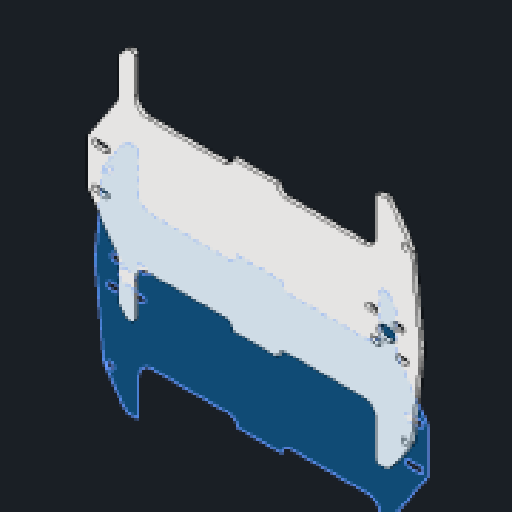
# Autodesk Inventor part: Aluminium Plate
Saved by Autodesk Inventor 2023.2 (Build 272271030, 271C)
## iProperties
Created: 2024-02-26
Part Number: Aluminium Plate
Material: Aluminum 6061
Document SubType Name: Modeling
Designer: robpl
Mass: 7.61954 g
Surface Area: 47.9052 cm^2
Volume: 2.82205 cm^3
Density: 2.7 g/cm^3
Appearance: Aluminum - Flat
Author: robpl
Autodesk Inventor part; units mm, degrees
ref_plane "YZ Plane" through (0, 0, 0) normal (1, 0, 0) x (0, 1, 0)
ref_plane "XZ Plane" through (0, 0, 0) normal (0, 1, 0) x (-1, 0, 0)
ref_plane "XY Plane" through (0, 0, 0) normal (0, 0, 1) x (1, 0, 0)
sketch "Sketch1" plane through (0, 0, 0) normal (0, 0, 1) x (1, 0, 0)
  arc A0 (49.1621, -12) -> (49.9853, -11.6297) centre (49.1621, -10.9) ccw projected
  arc A1 (49.9853, -11.6297) -> (61.3442, 6.3785) centre (0.77, 32) ccw projected
  arc A2 (61.3442, 6.3785) -> (60.2122, 9.0273) centre (59.5022, 7.1576) ccw projected
  arc A3 (61.2196, 14.348) -> (60.2122, 9.0273) centre (61.1884, 11.5982) ccw projected
  arc A4 (61.2196, 14.348) -> (63.2363, 16.5025) centre (61.2423, 16.3479) ccw projected
  line L0 (63.2363, 16.5025) -> (62.0377, 31.9587) projected
  line L1 (62.0377, 31.9587) -> (63.3538, 47.486) projected
  arc A5 (63.3538, 47.486) -> (61.2883, 49.6536) centre (61.3609, 47.6549) ccw projected
  arc A6 (60.2122, 54.9727) -> (61.2883, 49.6536) centre (61.1884, 52.4018) ccw projected
  arc A7 (60.2122, 54.9727) -> (61.3442, 57.6215) centre (59.5022, 56.8424) ccw projected
  arc A8 (61.3442, 57.6215) -> (49.9853, 75.6297) centre (0.77, 32) ccw projected
  arc A9 (49.9853, 75.6297) -> (49.1621, 76) centre (49.1621, 74.9) ccw projected
  line L2 (46.6, 76) -> (49.1621, 76) projected
  arc A10 (46.6, 76) -> (45.5, 74.9) centre (46.6, 74.9) ccw projected
  line L3 (45.5, 62) -> (45.5, 74.9) projected
  arc A11 (40.5, 57) -> (45.5, 62) centre (40.5, 62) ccw projected
  line L4 (11.3595, 57) -> (40.5, 57) projected
  arc A12 (8.3595, 60) -> (11.3595, 57) centre (11.3595, 60) ccw projected
  line L5 (-8.3595, 60) -> (8.3595, 60) projected
  arc A13 (-11.3595, 57) -> (-8.3595, 60) centre (-11.3595, 60) ccw projected
  line L6 (-40.5, 57) -> (-11.3595, 57) projected
  arc A14 (-45.5, 62) -> (-40.5, 57) centre (-40.5, 62) ccw projected
  line L7 (-45.5, 74.9) -> (-45.5, 62) projected
  arc A15 (-45.5, 74.9) -> (-46.6, 76) centre (-46.6, 74.9) ccw projected
  line L8 (-47.6221, 76) -> (-46.6, 76) projected
  arc A16 (-47.6221, 76) -> (-48.4453, 75.6297) centre (-47.6221, 74.9) ccw projected
  arc A17 (-48.4453, 75.6297) -> (-50.9534, 72.6248) centre (0.77, 32) ccw projected
  arc A18 (-50.9534, 72.6248) -> (-51.1884, 71.9454) centre (-50.0884, 71.9454) ccw projected
  line L9 (-51.1884, 71.9454) -> (-51.1884, 59.7084) projected
  arc A19 (-52.0225, 56.9433) -> (-51.1884, 59.7084) centre (-56.1884, 59.7084) ccw projected
  line L10 (-52.0225, 56.9433) -> (-62.4995, 41.1591) projected
  arc A20 (-62.4995, 41.1591) -> (-63, 39.5) centre (-60, 39.5) ccw projected
  line L11 (-63, 39.5) -> (-63, 24.5) projected
  arc A21 (-63, 24.5) -> (-62.4995, 22.8409) centre (-60, 24.5) ccw projected
  line L12 (-62.4995, 22.8409) -> (-52.0225, 7.0567) projected
  arc A22 (-51.1884, 4.2916) -> (-52.0225, 7.0567) centre (-56.1884, 4.2916) ccw projected
  line L13 (-51.1884, 4.2916) -> (-51.1884, -7.9454) projected
  arc A23 (-51.1884, -7.9454) -> (-50.9534, -8.6248) centre (-50.0884, -7.9454) ccw projected
  arc A24 (-50.9534, -8.6248) -> (-48.4453, -11.6297) centre (0.77, 32) ccw projected
  arc A25 (-48.4453, -11.6297) -> (-47.6221, -12) centre (-47.6221, -10.9) ccw projected
  line L14 (-46.6, -12) -> (-47.6221, -12) projected
  arc A26 (-46.6, -12) -> (-45.5, -10.9) centre (-46.6, -10.9) ccw projected
  line L15 (-45.5, 2) -> (-45.5, -10.9) projected
  arc A27 (-40.5, 7) -> (-45.5, 2) centre (-40.5, 2) ccw projected
  line L16 (-11.3595, 7) -> (-40.5, 7) projected
  arc A28 (-8.3595, 4) -> (-11.3595, 7) centre (-11.3595, 4) ccw projected
  line L17 (-8.3595, 4) -> (8.3595, 4) projected
  arc A29 (11.3595, 7) -> (8.3595, 4) centre (11.3595, 4) ccw projected
  line L18 (40.5, 7) -> (11.3595, 7) projected
  arc A30 (45.5, 2) -> (40.5, 7) centre (40.5, 2) ccw projected
  line L19 (45.5, -10.9) -> (45.5, 2) projected
  arc A31 (45.5, -10.9) -> (46.6, -12) centre (46.6, -10.9) ccw projected
  line L20 (49.1621, -12) -> (46.6, -12) projected
  line L21 (56.1569, 23.8431) -> (54.1569, 23.8431) projected
  arc A32 (54.1569, 28.8431) -> (54.1569, 23.8431) centre (54.1569, 26.3431) ccw projected
  line L22 (54.1569, 28.8431) -> (56.1569, 28.8431) projected
  arc A33 (56.1569, 23.8431) -> (56.1569, 28.8431) centre (56.1569, 26.3431) ccw projected
  line L23 (42.8431, 40.1569) -> (44.8431, 40.1569) projected
  arc A34 (44.8431, 35.1569) -> (44.8431, 40.1569) centre (44.8431, 37.6569) ccw projected
  line L24 (44.8431, 35.1569) -> (42.8431, 35.1569) projected
  arc A35 (42.8431, 40.1569) -> (42.8431, 35.1569) centre (42.8431, 37.6569) ccw projected
  arc A36 (45.0797, 30.2574) -> (46.0569, 31.4695) centre (45.0797, 31.2574) ccw projected
  arc A37 (48.5, 34.5) -> (46.0569, 31.4695) centre (48.5, 32) ccw projected
  line L25 (48.5, 34.5) -> (49.3223, 34.5) projected
  arc A38 (49.3223, 34.5) -> (50.2996, 35.7122) centre (49.3223, 35.5) ccw projected
  arc A39 (52.7426, 38.7426) -> (50.2996, 35.7122) centre (52.7426, 36.2426) ccw projected
  line L26 (52.7426, 38.7426) -> (54.7426, 38.7426) projected
  arc A40 (54.7426, 33.7426) -> (54.7426, 38.7426) centre (54.7426, 36.2426) ccw projected
  line L27 (54.7426, 33.7426) -> (53.9203, 33.7426) projected
  arc A41 (53.9203, 33.7426) -> (52.9431, 32.5305) centre (53.9203, 32.7426) ccw projected
  arc A42 (50.5, 29.5) -> (52.9431, 32.5305) centre (50.5, 32) ccw projected
  line L28 (50.5, 29.5) -> (49.6777, 29.5) projected
  arc A43 (49.6777, 29.5) -> (48.7004, 28.2878) centre (49.6777, 28.5) ccw projected
  arc A44 (46.2574, 25.2574) -> (48.7004, 28.2878) centre (46.2574, 27.7574) ccw projected
  line L29 (46.2574, 25.2574) -> (44.2574, 25.2574) projected
  arc A45 (44.2574, 30.2574) -> (44.2574, 25.2574) centre (44.2574, 27.7574) ccw projected
  line L30 (44.2574, 30.2574) -> (45.0797, 30.2574) projected
  arc A46 (-56, 22) -> (-56, 27) centre (-56, 24.5) ccw projected
  line L31 (-56, 22) -> (-60, 22) projected
  arc A47 (-60, 27) -> (-60, 22) centre (-60, 24.5) ccw projected
  line L32 (-60, 27) -> (-56, 27) projected
  line L33 (-56, 37) -> (-60, 37) projected
  arc A48 (-60, 42) -> (-60, 37) centre (-60, 39.5) ccw projected
  line L34 (-60, 42) -> (-56, 42) projected
  arc A49 (-56, 37) -> (-56, 42) centre (-56, 39.5) ccw projected
  arc A50 (63.4897, 12.2028) -> (63.5375, 12.619) centre (62.4407, 12.5339) ccw projected
  line L35 (63.5375, 12.619) -> (63.2363, 16.5025) projected
  arc A51 (61.2196, 14.348) -> (63.2363, 16.5025) centre (61.2423, 16.3479) ccw projected
  arc A52 (61.2196, 14.348) -> (60.2122, 9.0273) centre (61.1884, 11.5982) ccw projected
  arc A53 (61.3442, 6.3785) -> (60.2122, 9.0273) centre (59.5022, 7.1576) ccw projected
  arc A54 (61.3442, 6.3785) -> (63.4897, 12.2028) centre (0.77, 32) ccw projected
  circle A55 centre (61.1884, 11.5982) radius 1.25 projected
  circle A56 centre (61.1884, 52.4018) radius 1.25 projected
  arc A57 (63.652, 51.0045) -> (63.6069, 51.4222) centre (62.5559, 51.0974) ccw projected
  arc A58 (63.6069, 51.4222) -> (61.3442, 57.6215) centre (0.77, 32) ccw projected
  arc A59 (60.2122, 54.9727) -> (61.3442, 57.6215) centre (59.5022, 56.8424) ccw projected
  arc A60 (60.2122, 54.9727) -> (61.2883, 49.6536) centre (61.1884, 52.4018) ccw projected
  arc A61 (63.3538, 47.486) -> (61.2883, 49.6536) centre (61.3609, 47.6549) ccw projected
  line L36 (63.3538, 47.486) -> (63.652, 51.0045) projected
  line L37 (54.7426, 37.4926) -> (52.7426, 37.4926) projected
  arc A62 (54.7426, 34.9926) -> (54.7426, 37.4926) centre (54.7426, 36.2426) ccw projected
  line L38 (52.7426, 34.9926) -> (54.7426, 34.9926) projected
  arc A63 (52.7426, 37.4926) -> (52.7426, 34.9926) centre (52.7426, 36.2426) ccw projected
  arc A64 (52.9431, 32.5305) -> (50.5, 34.5) centre (50.5, 32) ccw projected
  arc A65 (53.9203, 33.7426) -> (52.9431, 32.5305) centre (53.9203, 32.7426) ccw projected
  line L39 (54.7426, 33.7426) -> (53.9203, 33.7426) projected
  arc A66 (54.7426, 33.7426) -> (54.7426, 38.7426) centre (54.7426, 36.2426) ccw projected
  line L40 (52.7426, 38.7426) -> (54.7426, 38.7426) projected
  arc A67 (52.7426, 38.7426) -> (50.2996, 35.7122) centre (52.7426, 36.2426) ccw projected
  arc A68 (49.3223, 34.5) -> (50.2996, 35.7122) centre (49.3223, 35.5) ccw projected
  line L41 (49.3223, 34.5) -> (50.5, 34.5) projected
  arc A69 (46.0569, 31.4695) -> (48.5, 29.5) centre (48.5, 32) ccw projected
  arc A70 (45.0797, 30.2574) -> (46.0569, 31.4695) centre (45.0797, 31.2574) ccw projected
  line L42 (44.2574, 30.2574) -> (45.0797, 30.2574) projected
  arc A71 (44.2574, 30.2574) -> (44.2574, 25.2574) centre (44.2574, 27.7574) ccw projected
  line L43 (46.2574, 25.2574) -> (44.2574, 25.2574) projected
  arc A72 (46.2574, 25.2574) -> (48.7004, 28.2878) centre (46.2574, 27.7574) ccw projected
  arc A73 (49.6777, 29.5) -> (48.7004, 28.2878) centre (49.6777, 28.5) ccw projected
  line L44 (49.6777, 29.5) -> (48.5, 29.5) projected
  line L45 (46.2574, 29.0074) -> (44.2574, 29.0074) projected
  arc A74 (46.2574, 26.5074) -> (46.2574, 29.0074) centre (46.2574, 27.7574) ccw projected
  line L46 (44.2574, 26.5074) -> (46.2574, 26.5074) projected
  arc A75 (44.2574, 29.0074) -> (44.2574, 26.5074) centre (44.2574, 27.7574) ccw projected
  arc A76 (54.1569, 28.8431) -> (54.1569, 23.8431) centre (54.1569, 26.3431) ccw projected
  line L47 (56.1569, 23.8431) -> (54.1569, 23.8431) projected
  arc A77 (56.1569, 23.8431) -> (56.1569, 28.8431) centre (56.1569, 26.3431) ccw projected
  line L48 (54.1569, 28.8431) -> (56.1569, 28.8431) projected
  line L49 (56.1569, 27.5931) -> (54.1569, 27.5931) projected
  arc A78 (56.1569, 25.0931) -> (56.1569, 27.5931) centre (56.1569, 26.3431) ccw projected
  line L50 (54.1569, 25.0931) -> (56.1569, 25.0931) projected
  arc A79 (54.1569, 27.5931) -> (54.1569, 25.0931) centre (54.1569, 26.3431) ccw projected
  arc A80 (44.8431, 35.1569) -> (44.8431, 40.1569) centre (44.8431, 37.6569) ccw projected
  line L51 (42.8431, 40.1569) -> (44.8431, 40.1569) projected
  arc A81 (42.8431, 40.1569) -> (42.8431, 35.1569) centre (42.8431, 37.6569) ccw projected
  line L52 (44.8431, 35.1569) -> (42.8431, 35.1569) projected
  line L53 (44.8431, 38.9069) -> (42.8431, 38.9069) projected
  arc A82 (44.8431, 36.4069) -> (44.8431, 38.9069) centre (44.8431, 37.6569) ccw projected
  line L54 (42.8431, 36.4069) -> (44.8431, 36.4069) projected
  arc A83 (42.8431, 38.9069) -> (42.8431, 36.4069) centre (42.8431, 37.6569) ccw projected
  line L55 (-56, 22) -> (-60, 22) projected
  arc A84 (-56, 22) -> (-56, 27) centre (-56, 24.5) ccw projected
  line L56 (-60, 27) -> (-56, 27) projected
  arc A85 (-60, 27) -> (-60, 22) centre (-60, 24.5) ccw projected
  line L57 (-60, 23.25) -> (-56, 23.25) projected
  arc A86 (-60, 25.75) -> (-60, 23.25) centre (-60, 24.5) ccw projected
  line L58 (-56, 25.75) -> (-60, 25.75) projected
  arc A87 (-56, 23.25) -> (-56, 25.75) centre (-56, 24.5) ccw projected
  arc A88 (-60, 42) -> (-60, 37) centre (-60, 39.5) ccw projected
  line L59 (-56, 37) -> (-60, 37) projected
  arc A89 (-56, 37) -> (-56, 42) centre (-56, 39.5) ccw projected
  line L60 (-60, 42) -> (-56, 42) projected
  line L61 (-60, 38.25) -> (-56, 38.25) projected
  arc A90 (-60, 40.75) -> (-60, 38.25) centre (-60, 39.5) ccw projected
  line L62 (-56, 40.75) -> (-60, 40.75) projected
  arc A91 (-56, 38.25) -> (-56, 40.75) centre (-56, 39.5) ccw projected
  point P0 (0, 0)
  point P1 (56.9489, 66.3148)
  point P2 (58.8517, 62.9872)
  point P3 (60.925, 8.5632)
  point P4 (62.8417, 15.1472)
  point P5 (56.9489, -2.3148)
  point P6 (58.8283, 1.0982)
  point P7 (58.6807, 0.8224)
  point P8 (58.7883, 1.2239)
  point P9 (56.8648, -2.3375)
extrude "Extrusion1" add sketch "Sketch1" along normal blind 1.6 contours L20 A31 L19 A30 L18 A29 L17 A28 L16 A27 L15 A26 L14 A25 A24 A23 L13 A22 L12 A21 L11 A20 L10 A19 L9 A18 A17 A16 L8 A15 L7 A14 L6 A13 L5 A12 L4 A11 L3 A10 L2 A9 A8 A7 A6 A5 L1 L0 A4 A3 A2 A1 A0 | A2 A3 A4 L35 A50 A54 | A5 A6 A7 A58 A57 L36 | L21 A32 L22 A33 | L23 A34 L24 A35 | A36 A69 L44 A43 A44 L29 A45 L30 | A38 A39 L26 A40 L27 A41 A64 L41 | L31 A47 L32 A46 | L33 A48 L34 A49
sketch "Sketch3" plane through (0, 0, 1.6) normal (0, 0, 1) x (1, 0, 0)
  arc A0 (49.9853, 75.6297) -> (49.1621, 76) centre (49.1621, 74.9) ccw projected
  line L0 (49.1621, 76) -> (46.6, 76) projected
  arc A1 (46.6, 76) -> (45.5, 74.9) centre (46.6, 74.9) ccw projected
  line L1 (45.5, 74.9) -> (45.5, 62) projected
  arc A2 (40.5, 57) -> (45.5, 62) centre (40.5, 62) ccw projected
  line L2 (40.5, 57) -> (11.3595, 57) projected
  arc A3 (8.3595, 60) -> (11.3595, 57) centre (11.3595, 60) ccw projected
  line L3 (8.3595, 60) -> (-8.3595, 60) projected
  arc A4 (-11.3595, 57) -> (-8.3595, 60) centre (-11.3595, 60) ccw projected
  line L4 (-11.3595, 57) -> (-40.5, 57) projected
  arc A5 (-45.5, 62) -> (-40.5, 57) centre (-40.5, 62) ccw projected
  line L5 (-45.5, 62) -> (-45.5, 74.9) projected
  arc A6 (-45.5, 74.9) -> (-46.6, 76) centre (-46.6, 74.9) ccw projected
  line L6 (-46.6, 76) -> (-47.6221, 76) projected
  arc A7 (-47.6221, 76) -> (-48.4453, 75.6297) centre (-47.6221, 74.9) ccw projected
  arc A8 (-48.4453, 75.6297) -> (-50.9534, 72.6248) centre (0.77, 32) ccw projected
  arc A9 (-50.9534, 72.6248) -> (-51.1884, 71.9454) centre (-50.0884, 71.9454) ccw projected
  line L7 (-51.1884, 71.9454) -> (-51.1884, 59.7084) projected
  arc A10 (-52.0225, 56.9433) -> (-51.1884, 59.7084) centre (-56.1884, 59.7084) ccw projected
  line L8 (-52.0225, 56.9433) -> (-62.4995, 41.1591) projected
  arc A11 (-62.4995, 41.1591) -> (-63, 39.5) centre (-60, 39.5) ccw projected
  line L9 (-63, 39.5) -> (-63, 24.5) projected
  arc A12 (-63, 24.5) -> (-62.4995, 22.8409) centre (-60, 24.5) ccw projected
  line L10 (-62.4995, 22.8409) -> (-52.0225, 7.0567) projected
  arc A13 (-51.1884, 4.2916) -> (-52.0225, 7.0567) centre (-56.1884, 4.2916) ccw projected
  line L11 (-51.1884, 4.2916) -> (-51.1884, -7.9454) projected
  arc A14 (-51.1884, -7.9454) -> (-50.9534, -8.6248) centre (-50.0884, -7.9454) ccw projected
  arc A15 (-50.9534, -8.6248) -> (-48.4453, -11.6297) centre (0.77, 32) ccw projected
  arc A16 (-48.4453, -11.6297) -> (-47.6221, -12) centre (-47.6221, -10.9) ccw projected
  line L12 (-47.6221, -12) -> (-46.6, -12) projected
  arc A17 (-46.6, -12) -> (-45.5, -10.9) centre (-46.6, -10.9) ccw projected
  line L13 (-45.5, -10.9) -> (-45.5, 2) projected
  arc A18 (-40.5, 7) -> (-45.5, 2) centre (-40.5, 2) ccw projected
  line L14 (-40.5, 7) -> (-11.3595, 7) projected
  arc A19 (-8.3595, 4) -> (-11.3595, 7) centre (-11.3595, 4) ccw projected
  line L15 (-8.3595, 4) -> (8.3595, 4) projected
  arc A20 (11.3595, 7) -> (8.3595, 4) centre (11.3595, 4) ccw projected
  line L16 (11.3595, 7) -> (40.5, 7) projected
  arc A21 (45.5, 2) -> (40.5, 7) centre (40.5, 2) ccw projected
  line L17 (45.5, 2) -> (45.5, -10.9) projected
  arc A22 (45.5, -10.9) -> (46.6, -12) centre (46.6, -10.9) ccw projected
  line L18 (46.6, -12) -> (49.1621, -12) projected
  arc A23 (49.1621, -12) -> (49.9853, -11.6297) centre (49.1621, -10.9) ccw projected
  arc A24 (49.9853, -11.6297) -> (63.4897, 12.2028) centre (0.77, 32) ccw projected
  arc A25 (63.4897, 12.2028) -> (63.5375, 12.619) centre (62.4407, 12.5339) ccw projected
  line L19 (63.5375, 12.619) -> (62.0377, 31.9587) projected
  line L20 (62.0377, 31.9587) -> (63.652, 51.0045) projected
  arc A26 (63.652, 51.0045) -> (63.6069, 51.4222) centre (62.5559, 51.0974) ccw projected
  arc A27 (63.6069, 51.4222) -> (49.9853, 75.6297) centre (0.77, 32) ccw projected
  arc A28 (44.8431, 36.4069) -> (44.8431, 38.9069) centre (44.8431, 37.6569) ccw projected
  line L21 (44.8431, 36.4069) -> (42.8431, 36.4069) projected
  arc A29 (42.8431, 38.9069) -> (42.8431, 36.4069) centre (42.8431, 37.6569) ccw projected
  line L22 (42.8431, 38.9069) -> (44.8431, 38.9069) projected
  arc A30 (56.1569, 25.0931) -> (56.1569, 27.5931) centre (56.1569, 26.3431) ccw projected
  line L23 (56.1569, 25.0931) -> (54.1569, 25.0931) projected
  arc A31 (54.1569, 27.5931) -> (54.1569, 25.0931) centre (54.1569, 26.3431) ccw projected
  line L24 (54.1569, 27.5931) -> (56.1569, 27.5931) projected
  arc A32 (-60, 25.75) -> (-60, 23.25) centre (-60, 24.5) ccw projected
  line L25 (-60, 25.75) -> (-56, 25.75) projected
  arc A33 (-56, 23.25) -> (-56, 25.75) centre (-56, 24.5) ccw projected
  line L26 (-56, 23.25) -> (-60, 23.25) projected
  arc A34 (-60, 40.75) -> (-60, 38.25) centre (-60, 39.5) ccw projected
  line L27 (-60, 40.75) -> (-56, 40.75) projected
  arc A35 (-56, 38.25) -> (-56, 40.75) centre (-56, 39.5) ccw projected
  line L28 (-56, 38.25) -> (-60, 38.25) projected
  circle A36 centre (61.1884, 52.4018) radius 1.25 projected
  circle A37 centre (61.1884, 11.5982) radius 1.25 projected
  arc A38 (46.2574, 26.5074) -> (46.2574, 29.0074) centre (46.2574, 27.7574) ccw projected
  line L29 (46.2574, 26.5074) -> (44.2574, 26.5074) projected
  arc A39 (44.2574, 29.0074) -> (44.2574, 26.5074) centre (44.2574, 27.7574) ccw projected
  line L30 (44.2574, 29.0074) -> (46.2574, 29.0074) projected
  arc A40 (50.5, 29.5) -> (50.5, 34.5) centre (50.5, 32) ccw projected
  line L31 (50.5, 29.5) -> (48.5, 29.5) projected
  arc A41 (48.5, 34.5) -> (48.5, 29.5) centre (48.5, 32) ccw projected
  line L32 (48.5, 34.5) -> (50.5, 34.5) projected
  arc A42 (54.7426, 34.9926) -> (54.7426, 37.4926) centre (54.7426, 36.2426) ccw projected
  line L33 (54.7426, 34.9926) -> (52.7426, 34.9926) projected
  arc A43 (52.7426, 37.4926) -> (52.7426, 34.9926) centre (52.7426, 36.2426) ccw projected
  line L34 (52.7426, 37.4926) -> (54.7426, 37.4926) projected
  line L35 (50.5, -2.9274) -> (50.5, 2)
  arc A44 (50.5, 2) -> (40.5, 12) centre (40.5, 2) ccw
  line L36 (40.5, 12) -> (11.3595, 12)
  arc A45 (11.3595, 12) -> (5.1145, 9) centre (11.3595, 4) ccw
  line L37 (5.1145, 9) -> (-5.1145, 9)
  arc A46 (-5.1145, 9) -> (-11.3595, 12) centre (-11.3595, 4) ccw
  line L38 (-11.3595, 12) -> (-40.5, 12)
  arc A47 (-40.5, 12) -> (-46.1884, 10.2245) centre (-40.5, 2) ccw
  line L39 (-46.1884, 10.2245) -> (-46.1884, 4.2916)
  arc A48 (-46.1884, 4.2916) -> (-47.8567, 9.8219) centre (-56.1884, 4.2916) ccw
  line L40 (-47.8567, 9.8219) -> (-58, 25.1034)
  line L41 (-58, 25.1034) -> (-58, 38.8966)
  line L42 (-58, 38.8966) -> (-47.8567, 54.1781)
  arc A49 (-47.8567, 54.1781) -> (-46.1884, 59.7084) centre (-56.1884, 59.7084) ccw
  line L43 (-46.1884, 59.7084) -> (-46.1884, 53.7755)
  arc A50 (-46.1884, 53.7755) -> (-40.5, 52) centre (-40.5, 62) ccw
  line L44 (-40.5, 52) -> (-11.3595, 52)
  arc A51 (-11.3595, 52) -> (-5.1145, 55) centre (-11.3595, 60) ccw
  line L45 (-5.1145, 55) -> (5.1145, 55)
  arc A52 (5.1145, 55) -> (11.3595, 52) centre (11.3595, 60) ccw
  line L46 (11.3595, 52) -> (40.5, 52)
  arc A53 (40.5, 52) -> (50.5, 62) centre (40.5, 62) ccw
  line L47 (50.5, 62) -> (50.5, 66.9274)
  arc A54 (58.6047, 50.6584) -> (50.5, 66.9274) centre (0.77, 32) ccw
  line L48 (58.6047, 50.6584) -> (57.0213, 31.9766)
  line L49 (57.0213, 31.9766) -> (58.493, 12.9987)
  arc A55 (50.5, -2.9274) -> (58.493, 12.9987) centre (0.77, 32) ccw
  line L50 (11.3595, 52) -> (8.3595, 52)
  line L51 (8.3595, 52) -> (-11.3595, 52)
  arc A56 (8.3595, 60) -> (11.3595, 57) centre (11.3595, 60) ccw projected
  line L52 (11.3595, 57) -> (-11.3595, 57)
  arc A57 (11.3595, 7) -> (8.3595, 4) centre (11.3595, 4) ccw projected
  line L53 (11.3595, 7) -> (-11.3595, 7)
  line L54 (11.3595, 12) -> (-11.3595, 12)
  circle A58 centre (61.1884, 11.5982) radius 3
  circle A59 centre (61.1884, 52.4018) radius 3
  line L55 (42.8431, 34.4069) -> (44.8431, 34.4069)
  arc A60 (44.8431, 34.4069) -> (44.8431, 40.9069) centre (44.8431, 37.6569) ccw
  line L56 (44.8431, 40.9069) -> (42.8431, 40.9069)
  arc A61 (42.8431, 40.9069) -> (42.8431, 34.4069) centre (42.8431, 37.6569) ccw
  arc A62 (46.2574, 24.5074) -> (46.2574, 31.0074) centre (46.2574, 27.7574) ccw
  line L57 (46.2574, 24.5074) -> (44.2574, 24.5074)
  arc A63 (44.2574, 31.0074) -> (44.2574, 24.5074) centre (44.2574, 27.7574) ccw
  line L58 (44.2574, 31.0074) -> (46.2574, 31.0074)
  line L59 (48.5, 27.5) -> (50.5, 27.5)
  arc A64 (50.5, 27.5) -> (50.5, 36.5) centre (50.5, 32) ccw
  line L60 (50.5, 36.5) -> (48.5, 36.5)
  arc A65 (48.5, 36.5) -> (48.5, 27.5) centre (48.5, 32) ccw
  line L61 (52.7426, 32.9926) -> (54.7426, 32.9926)
  arc A66 (54.7426, 32.9926) -> (54.7426, 39.4926) centre (54.7426, 36.2426) ccw
  line L62 (54.7426, 39.4926) -> (52.7426, 39.4926)
  arc A67 (52.7426, 39.4926) -> (52.7426, 32.9926) centre (52.7426, 36.2426) ccw
  line L63 (54.1569, 23.0931) -> (56.1569, 23.0931)
  arc A68 (56.1569, 23.0931) -> (56.1569, 29.5931) centre (56.1569, 26.3431) ccw
  line L64 (56.1569, 29.5931) -> (54.1569, 29.5931)
  arc A69 (54.1569, 29.5931) -> (54.1569, 23.0931) centre (54.1569, 26.3431) ccw
  arc A70 (40.5, 57) -> (45.5, 62) centre (40.5, 62) ccw projected
  line L65 (11.3595, 7) -> (40.5, 7) projected
  line L66 (40.5, 7) -> (61.4182, 8.607)
  line L67 (40.5, 12) -> (58.7938, 13.4054)
  line L68 (40.5, 57) -> (61.4182, 55.393)
  line L69 (40.5, 52) -> (58.6006, 50.6094)
  arc A71 (-60, 42.75) -> (-60, 36.25) centre (-60, 39.5) ccw
  line L70 (-60, 42.75) -> (-56, 42.75)
  arc A72 (-56, 36.25) -> (-56, 42.75) centre (-56, 39.5) ccw
  line L71 (-56, 36.25) -> (-60, 36.25)
  arc A73 (-60, 27.75) -> (-60, 21.25) centre (-60, 24.5) ccw
  line L72 (-60, 27.75) -> (-56, 27.75)
  arc A74 (-56, 21.25) -> (-56, 27.75) centre (-56, 24.5) ccw
  line L73 (-56, 21.25) -> (-60, 21.25)
  arc A75 (-40.5, 7) -> (-45.5, 2) centre (-40.5, 2) ccw projected
  line L74 (-40.5, 7) -> (-61.8539, 21.8306)
  line L75 (-52.0225, 56.9433) -> (-62.4995, 41.1591) projected
  arc A76 (-45.5, 62) -> (-40.5, 57) centre (-40.5, 62) ccw projected
  line L76 (-61.8082, 42.2005) -> (-40.5, 57)
  line L77 (-38.934, 12) -> (-53.6699, 22.2343)
  line L78 (-38.9339, 52) -> (-53.6697, 41.7654)
  point P0 (0, 0)
  point P1 (62.3197, 55.1803)
  point P2 (62.3197, 8.8197)
  point P3 (11.3595, 12)
  point P4 (58.4634, 13.38)
  point P5 (57.6808, 23.4726)
  point P6 (51.1374, 27.5454)
  point P7 (49.4972, 27.5)
  point P8 (44.1116, 31.0041)
  point P9 (44.6978, 34.4069)
  point P10 (47.8626, 36.4546)
  point P11 (49.5028, 36.5)
  point P12 (57.5252, 37.9219)
  point P13 (-58, 36.25)
  point P14 (-58, 27.75)
  point P15 (-61.8075, 21.7984)
  point P16 (-61.8082, 42.2005)
  dimension "d17" = 5
  dimension "d20" = 2
  dimension "d21" = 2
  dimension "d22" = 2
  dimension "d23" = 2
  dimension "d24" = 2
  dimension "d25" = 2
  dimension "d26" = 2
  dimension "d27" = 5
  constraints: 84 end point, 59 point on circle, 27 centre point, 8 tangent, 5 parallel, 4 point on line, 2 collinear, 1 equal length, 1 horizontal, 52 other
  measures "d17" distance between parallel lines of L17 L35
  measures "d20" distance between parallel lines of L21 L55
  measures "d21" radial gap between concentric circles of A38 A62
  measures "d22" radial gap between concentric circles of A41 A65
  measures "d23" radial gap between concentric circles of A43 A67
  measures "d24" distance between parallel lines of L23 L63
  measures "d25" distance between parallel lines of L28 L71
  measures "d26" distance between parallel lines of L26 L73
  measures "d27" distance between parallel lines of L77 L74
extrude "Extrusion3" cut sketch "Sketch3" against normal blind 1.6 contours A27 A59 L68 A54 L47 A53 A2 L1 A1 L0 A0 | L68 A53 L47 A54 | L48 A66 L62 A67 L60 A65 A60 L56 A61 L55 A63 L57 A62 L59 A64 A69 L63 A68 L49 L67 L36 L54 L38 L77 A74 L72 L41 L71 A72 L78 L44 L51 L50 L46 L69 | L52 A4 L3 A3 | A24 A23 L18 A22 L17 A21 L66 A44 L35 A55 A58 | L76 A50 L43 A49 L42 L8 A10 L7 A9 A8 A7 L6 A6 L5 A5 | A55 L35 A44 L66 | L76 L42 A49 L43 A50 | A20 L15 A19 L53 | A18 L13 A17 L12 A16 A15 A14 L11 A13 L10 L74 L40 A48 L39 A47 | A47 L39 A48 L40 L74
body "Solid1"
